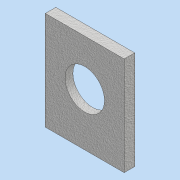
# Autodesk Inventor part: Uchwyt silnika krokowego osi Z - płaski
Saved by Autodesk Inventor 2018 (Build 220112000, 112)
## iProperties
Created: 2019-02-02
Part Number: Uchwyt silnika krokowego osi Z - płaski
Material: Ogólny
Document SubType Name: Modeling
Designer: Dawid
Density: 1 g/cm^3
Appearance: Aluminium odlewane
Author: Dawid
Autodesk Inventor part; units mm, degrees
ref_plane "YZ Plane" through (0, 0, 0) normal (1, 0, 0) x (0, 1, 0)
ref_plane "XZ Plane" through (0, 0, 0) normal (0, 1, 0) x (-1, 0, 0)
ref_plane "XY Plane" through (0, 0, 0) normal (0, 0, 1) x (1, 0, 0)
sketch "Szkic1" plane through (0, 0, 0) normal (0, 1, 0) x (-1, 0, 0)
  line L0 (-30, 37.5) -> (30, 37.5)
  line L1 (30, 37.5) -> (30, -37.5)
  line L2 (30, -37.5) -> (-30, -37.5)
  line L3 (-30, -37.5) -> (-30, 37.5)
  line L4 (-30, 37.5) -> (30, -37.5) construction
  line L5 (30, 37.5) -> (-30, -37.5) construction
  point P0 (0, 0)
  dimension "d0" = 60
  dimension "d1" = 75
  constraints: 12 end point, 2 midpoint, 2 parallel, 1 horizontal, 1 perpendicular
  measures "d0" distance of L1.end L2.end
  measures "d1" distance of L0.end L1.end
extrude "Wyciągnięcie proste1" add sketch "Szkic1" along normal blind 8
sketch "Szkic2" plane through (0, 8, 0) normal (0, 1, 0) x (1, 0, 0)
  line L0 (-30, -37.5) -> (30, -37.5) projected
  line L1 (0, -37.5) -> (0, -2.5)
  circle A0 centre (0, -2.5) radius 20
  point P0 (0, 0)
  dimension "d4" = 35
  dimension "d5" = 40
  constraints: 2 end point, 1 centre point, 1 coincident, 1 midpoint, 1 vertical
  measures "d4" distance of L1.start L1.end
  measures "d5" diameter of A0
extrude "Wyciągnięcie proste2" cut sketch "Szkic2" against normal blind 2
sketch "Szkic3" plane through (0, 6, 2.5) normal (0, 1, 0) x (1, 0, 0)
  circle A0 centre (0, 0) radius 20 projected
  circle A1 centre (0, 0) radius 5
  point P0 (0, 2.5)
  dimension "d8" = 10
  constraints: 1 centre point, 1 coincident
  measures "d8" diameter of A1
extrude "Wyciągnięcie proste3" cut sketch "Szkic3" against normal up to next contours A1
sketch "Szkic4" plane through (0, 0, 0) normal (0, -1, 0) x (1, 0, 0)
  circle A0 centre (0, 2.5) radius 5 projected
  circle A1 centre (0, 2.5) radius 15
  point P0 (0, 0)
  dimension "d11" = 30
  constraints: 1 centre point, 1 coincident
  measures "d11" diameter of A1
extrude "Wyciągnięcie proste4" cut sketch "Szkic4" against normal up to next
